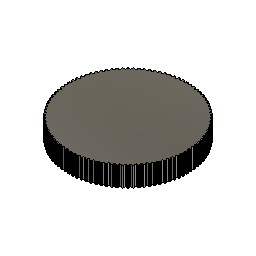
gear_96z (Autodesk Fusion 360 design; units mm, degrees)
Autodesk Fusion 360 part; units mm, degrees
sketch "Sketch1" plane through (0, 0, 0) normal (0, 0, 1) x (1, 0, 0) in component "gt2 pulley"
  circle A0 centre (0, 0) radius 30.5577 construction
  circle A1 centre (0, 0) radius 29.5537 construction
  line L0 (0, 0) -> (0, 30.5577) construction
  line L1 (0, 0) -> (0.9998, 30.5414) construction
  line L2 (0, 0) -> (1.4042, 30.5255) construction
  circle A2 centre (0, 0) radius 30.3037 construction
  arc A3 (0.3979, 30.1682) -> (0.4771, 29.8692) centre (1.3925, 30.2717) ccw
  circle A4 centre (0, 0) radius 30.1537 construction
  arc A5 (0.2498, 30.3027) -> (0, 30.3037) centre (0, 0) ccw
  arc A6 (0.3979, 30.1682) -> (0.2498, 30.3027) centre (0.2487, 30.1527) ccw
  arc A7 (0.4771, 29.8692) -> (0.967, 29.5379) centre (0.9851, 30.0926) ccw
  arc A8 (0, 30.3037) -> (-0.2498, 30.3027) centre (0, 0) ccw
  arc A9 (-0.2498, 30.3027) -> (-0.3979, 30.1682) centre (-0.2487, 30.1527) ccw
  arc A10 (-0.4771, 29.8692) -> (-0.3979, 30.1682) centre (-1.3925, 30.2717) ccw
  arc A11 (-0.9673, 29.5379) -> (-0.4771, 29.8692) centre (-0.9851, 30.0926) ccw
  arc A12 (0.967, 29.5379) -> (-0.967, 29.5379) centre (0, 0) ccw
  point P0 (1.3925, 30.2717)
  point P1 (0, 30.3037)
  dimension "d18" = 61.1155
  dimension "d19" = 1.875
  dimension "d22" = 1.004
  dimension "d24" = 0.75
  dimension "d26" = 1
  dimension "d27" = 0.15
  dimension "d28" = 0.15
  dimension "d47" = 0.555
  dimension "d52" = 3.812
  constraint coincident A0.centre A1.centre
  constraint coincident A0 L0.end
  constraint vertical L0
  constraint coincident A0 L1.end
  constraint coincident A0 L2.end
  constraint concentric A1 A2
  constraint coincident A1 A7.end
  constraint coincident L1 A7.end
  constraint coincident A2 P0
  constraint coincident L2 P0
  constraint coincident P0 A3.centre
  constraint coincident A2 P1
  constraint coincident L0 P1
  constraint concentric A2 A4
  constraint coincident P1 A5.end
  constraint coincident A4 A6.centre
  constraint coincident A3.start A6.start
  constraint tangent A3 A6
  constraint tangent A3 A7
  constraint symmetric L0 A7.end A12.end
  constraint symmetric L0 A3.start A9.end
  constraint symmetric L0 A3.end A10.start
  constraint symmetric L0 A3 A10
  constraint symmetric L0 A5.start A8.end
  constraint symmetric L0 P1 A5.end
  constraint symmetric L0 A5 A8
  constraint symmetric L0 A6 A9
  constraint symmetric L0 A7 A11
  constraint coincident A1 A11.start
  constraint tangent A1 A7
  constraint coincident L1 A7.centre
  measures "d18" diameter of A0
  measures "d19" angle of L0 L1
  measures "d22" distance of A0 A1
  measures "d24" distance of A1 A2
  measures "d26" radius of A3
  measures "d27" distance of A2 A4
  measures "d28" radius of A6
  measures "d47" radius of A7
extrude "Extrude1" add sketch "Sketch1" along normal blind 10 makes body 1
pattern_circular "C-Pattern1" count 96 over 360 about axis through (0, 0, 1.75) along (0, 0, 1) of bodies 1 makes body 2 at (-1.1818, 29.5301, 3.3333) makes body 3 at (-4.6023, 29.1932, 6.6667) makes body 4 at (-6.2919, 28.8762, 6.6667) makes body 5 at (-8.167, 28.4029, 6.6667) makes body 6 at (-8.7845, 28.218, 3.3333) makes body 7 at (-11.4091, 27.2627, 6.6667) makes body 8 at (-13.1678, 26.4582, 6.6667) makes body 9 at (-14.1207, 25.9621, 3.3333) makes body 10 at (-16.5086, 24.5131, 6.6667) makes body 11 at (-18.0765, 23.3809, 6.6667) makes body 12 at (-18.9144, 22.7084, 3.3333) makes body 13 at (-20.9736, 20.8214, 6.6667) makes body 14 at (-22.2905, 19.4051, 6.6667) makes body 15 at (-23.7699, 17.5617, 6.6667) makes body 16 at (-24.6327, 16.3296, 6.6667) makes body 17 at (-25.21, 15.4234, 3.3333) makes body 18 at (-26.1647, 13.7416, 6.6667) makes body 19 at (-27.0074, 12.0009, 3.3333) makes body 20 at (-28.0198, 9.3977, 6.6667) makes body 21 at (-28.3428, 8.3731, 3.3333) makes body 22 at (-29.0067, 5.66, 6.6667) makes body 23 at (-29.3896, 3.1103, 6.6667) makes body 24 at (-29.4317, 2.6828, 3.3333) makes body 25 at (-29.5536, -0.1077, 6.6667) makes body 26 at (-29.5301, -1.1818, 3.3333) makes body 27 at (-29.1932, -4.6023, 6.6667) makes body 28 at (-28.8762, -6.2919, 6.6667) makes body 29 at (-28.5187, -7.753, 6.6667) makes body 30 at (-27.9505, -9.6016, 6.6667) makes body 31 at (-27.0073, -12.0013, 6.6667) makes body 32 at (-26.1646, -13.7419, 6.6667) makes body 33 at (-25.9621, -14.1207, 3.3333) makes body 34 at (-24.5131, -16.5086, 6.6667) makes body 35 at (-23.3809, -18.0765, 6.6667) makes body 36 at (-22.7084, -18.9144, 3.3333) makes body 37 at (-20.3588, -21.423, 6.6667) makes body 38 at (-20.0453, -21.7166, 3.3333) makes body 39 at (-18.582, -22.9811, 3.3333) makes body 40 at (-16.3296, -24.6327, 6.6667) makes body 41 at (-14.1204, -25.9622, 6.6667) makes body 42 at (-13.7416, -26.1647, 6.6667) makes body 43 at (-11.2102, -27.3451, 6.6667) makes body 44 at (-9.3977, -28.0198, 6.6667) makes body 45 at (-7.545, -28.5744, 6.6667) makes body 46 at (-5.66, -29.0067, 6.6667) makes body 47 at (-3.7508, -29.3148, 6.6667) makes body 48 at (-2.6828, -29.4317, 3.3333) makes body 49 at (0.1077, -29.5536, 6.6667) makes body 50 at (2.6831, -29.4317, 6.6667) makes body 51 at (4.6023, -29.1932, 6.6667) makes body 52 at (6.2919, -28.8762, 6.6667) makes body 53 at (7.753, -28.5187, 6.6667) makes body 54 at (9.6016, -27.9505, 6.6667) makes body 55 at (12.0013, -27.0073, 6.6667) makes body 56 at (13.7419, -26.1646, 6.6667) makes body 57 at (14.1207, -25.9621, 3.3333) makes body 58 at (15.7885, -24.9829, 3.3333) makes body 59 at (18.0765, -23.3809, 6.6667) makes body 60 at (18.9144, -22.7084, 3.3333) makes body 61 at (20.9736, -20.8214, 6.6667) makes body 62 at (21.7166, -20.0453, 3.3333) makes body 63 at (22.9811, -18.582, 3.3333) makes body 64 at (24.6327, -16.3296, 6.6667) makes body 65 at (25.21, -15.4234, 3.3333) makes body 66 at (26.1647, -13.7416, 6.6667) makes body 67 at (27.0074, -12.0009, 3.3333) makes body 68 at (28.0198, -9.3977, 6.6667) makes body 69 at (28.3428, -8.3731, 3.3333) makes body 70 at (29.0067, -5.66, 6.6667) makes body 71 at (29.3896, -3.1103, 6.6667) makes body 72 at (29.4317, -2.6828, 3.3333) makes body 73 at (29.5536, 0.1077, 6.6667) makes body 74 at (29.5301, 1.1818, 3.3333) makes body 75 at (29.1932, 4.6023, 6.6667) makes body 76 at (29.1232, 5.0261, 3.3333) makes body 77 at (28.5187, 7.753, 6.6667) makes body 78 at (27.9505, 9.6016, 6.6667) makes body 79 at (27.0073, 12.0013, 6.6667) makes body 80 at (26.1646, 13.7419, 6.6667) makes body 81 at (25.9621, 14.1207, 3.3333) makes body 82 at (24.5131, 16.5086, 6.6667) makes body 83 at (23.8968, 17.3887, 3.3333) makes body 84 at (21.7163, 20.0456, 6.6667) makes body 85 at (20.8214, 20.9736, 6.6667) makes body 86 at (19.4051, 22.2905, 6.6667) makes body 87 at (18.582, 22.9811, 3.3333) makes body 88 at (15.7882, 24.9831, 6.6667) makes body 89 at (14.1204, 25.9622, 6.6667) makes body 90 at (13.7416, 26.1647, 6.6667) makes body 91 at (12.0009, 27.0074, 3.3333) makes body 92 at (9.3977, 28.0198, 6.6667) makes body 93 at (7.545, 28.5744, 6.6667) makes body 94 at (5.66, 29.0067, 6.6667) makes body 95 at (3.7508, 29.3148, 6.6667) makes body 96 at (2.6828, 29.4317, 3.3333)
sketch "Sketch2" plane through (0, 0, 10) normal (0, 0, 1) x (-1, 0, 0)
  arc A0 (-10.074, -28.4393) -> (-9.9771, -28.6142) centre (-9.9277, -28.4726) ccw
  arc A1 (-9.9771, -28.6142) -> (-9.5039, -28.7749) centre (0, 0) ccw
  arc A2 (-9.5039, -28.7749) -> (-9.3205, -28.6951) centre (-9.4568, -28.6325) ccw
  arc A3 (-9.1494, -28.4374) -> (-9.3205, -28.6951) centre (-8.4119, -29.1128) ccw
  arc A4 (-8.579, -28.2812) -> (-9.1494, -28.4374) centre (-8.7401, -28.8123) ccw
  arc A5 (-10.4103, -27.6595) -> (-8.579, -28.2812) centre (0, 0) ccw
  arc A6 (-10.0529, -28.1307) -> (-10.4103, -27.6595) centre (-10.6058, -28.179) ccw
  arc A7 (-10.074, -28.4393) -> (-10.0529, -28.1307) centre (-11.0491, -28.2176) ccw
  circle A8 centre (0, 0) radius 29.5537
  constraint coincident A1.centre A5.centre
extrude "Extrude2" add sketch "Sketch2" against normal blind 10 contours A5 A8 bodies 1 2 3 4 5 6 7 8 9 10 11 12 13 14 15 16 17 18 19 20 21 22 23 24 25 26 27 28 29 30 31 32 33 34 35 36 37 38 39 40 41 42 43 44 45 46 47 48 49 50 51 52 53 54 55 56 57 58 59 60 61 62 63 64 65 66 67 68 69 70 71 72 73 74 75 76 77 78 79 80 81 82 83 84 85 86 87 88 89 90 91 92 93 94 95 96
extrude "Extrude4" [suppressed] in component "gt2 pulley"
pattern_circular "C-Pattern7" [suppressed] in component "gt2 pulley"
extrude "Extrude3" [suppressed] in component "gt2 pulley"
pattern_circular "C-Pattern6" [suppressed] in component "gt2 pulley"
extrude "Extrude2'" [suppressed] in component "gt2 pulley"
pattern_circular "C-Pattern5" [suppressed] in component "gt2 pulley"
extrude "Extrude1'" [suppressed] in component "gt2 pulley"
pattern_circular "C-Pattern4" [suppressed] in component "gt2 pulley"
pattern_circular "C-Pattern3" [suppressed] in component "gt2 pulley"
pattern_circular "C-Pattern2" [suppressed] in component "gt2 pulley"
pattern_circular "C-Pattern1'" [suppressed] in component "gt2 pulley"
copy_body "Body->Comp1" [suppressed] in component "Component"
copy_body "Body->Comp2" [suppressed] in component "Component'"
copy_body "Body->Comp3" [suppressed] in component "Component''"
copy_body "Body->Comp4" [suppressed] in component "Component'''"
copy_body "Body->Comp5" [suppressed] in component "Component''''"
copy_body "Body->Comp6" [suppressed] in component "Component'''''"
copy_body "Body->Comp7" [suppressed] in component "Component''''''"
copy_body "Body->Comp8" [suppressed] in component "Component'''''''"
copy_body "Body->Comp9" [suppressed] in component "Component''''''''"
copy_body "Body->Comp10" [suppressed] in component "Component'''''''''"
copy_body "Body->Comp11" [suppressed] in component "Component''''''''''"
copy_body "Body->Comp12" [suppressed] in component "Component'''''''''''"
copy_body "Body->Comp13" [suppressed] in component "Component''''''''''''"
copy_body "Body->Comp14" [suppressed] in component "Component'''''''''''''"
copy_body "Body->Comp15" [suppressed] in component "Component''''''''''''''"
copy_body "Body->Comp16" [suppressed] in component "Component'''''''''''''''"
copy_body "Body->Comp17" [suppressed] in component "Component''''''''''''''''"
copy_body "Body->Comp18" [suppressed] in component "Component'''''''''''''''''"
copy_body "Body->Comp19" [suppressed] in component "Component''''''''''''''''''"
copy_body "Body->Comp20" [suppressed] in component "Component'''''''''''''''''''"
component "gt2 pulley" placed x (1, 0, 0) y (0, 1, 0) z (0, 0, 1) at (0, 0, 0)
equation "NumTeeth = 96" comment "min 20"
equation "ToothPitch = 2 mm"
equation "PullyDia = NumTeeth * ToothPitch / PI"
equation "ToothAng = ( ( 360 / NumTeeth ) * 1 deg )"
equation "TransOffsetAngle = ToothAng * 0.2"
equation "Sholulder_Radius = 0.15 mm"
equation "Root_Radius = 0.555 mm"
equation "TransRadius = 1 mm"
equation "ToolHeight = 0.75 mm"
equation "PLD = 0.254 mm"
equation "d18 = PullyDia"
equation "d19 = ToothAng / 2"
equation "d22 = PLD + ToolHeight"
equation "d24 = ToolHeight"
equation "d26 = TransRadius"
equation "d27 = Sholulder_Radius"
equation "d31 = NumTeeth"
equation "d33 = NumTeeth"
equation "d35 = NumTeeth"
equation "d37 = NumTeeth"
equation "d41 = NumTeeth"
equation "d45 = NumTeeth"
equation "d47 = Root_Radius"
equation "d50 = NumTeeth"
